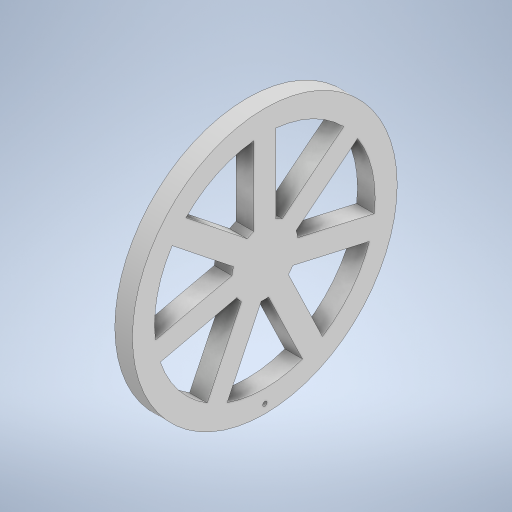
# Autodesk Inventor part: Langbektang houder
Saved by Autodesk Inventor 2023.2 (Build 272271000, 271)
## iProperties
Created: 2020-09-09
Part Number: Langbektang houder
Material: Generic
Document SubType Name: Modeling
Designer: nathan.bollaert
Density: 1 g/cm^3
Appearance: Default
Author: nathan.bollaert
Autodesk Inventor part; units mm, degrees
ref_plane "YZ Plane" through (0, 0, 0) normal (1, 0, 0) x (0, 1, 0)
ref_plane "XZ Plane" through (0, 0, 0) normal (0, 1, 0) x (-1, 0, 0)
ref_plane "XY Plane" through (0, 0, 0) normal (0, 0, 1) x (1, 0, 0)
sketch "Sketch1" plane through (0, 0, 0) normal (1, 0, 0) x (0, 1, 0)
  circle A0 centre (0, 0) radius 30
  dimension "d228" = 60
  constraints: 1 centre point, 1 coincident
  measures "d228" diameter of A0
extrude "Extrusion1" add sketch "Sketch1" along normal blind 4
sketch "Sketch2" plane through (4, 0, 0) normal (1, 0, 0) x (0, 0, -1)
  circle A0 centre (0, -28) radius 0.5
  point P0 (0, 0)
  dimension "d231" = 1
  dimension "d233" = 28
  constraints: 1 centre point, 1 vertical alignment
  measures "d231" diameter of A0
  measures "d233" distance of point (0, 0) A0.centre
hole "Hole1" at (4, -28, 0) direction (-1, 0, 0) diameter 1 end through all
sketch "Sketch3" plane through (4, 0, 0) normal (1, 0, 0) x (0, 0, -1)
  circle A0 centre (0, 0) radius 30 projected
  line L0 (-2.5, 25) -> (2.5, 25)
  line L1 (0, -42) -> (0, 42) projected
  circle A1 centre (0, 0) radius 7.5
  line L2 (2.5, 25) -> (2.5, 7.0711)
  line L3 (-2.5, 7.0711) -> (-2.5, 25)
  circle A2 centre (0, 0) radius 25
  line L4 (-17.9871, 17.5418) -> (-3.9697, 6.3633)
  line L5 (-21.1045, 13.6327) -> (-17.9871, 17.5418)
  line L6 (-7.0871, 2.4542) -> (-21.1045, 13.6327)
  line L7 (-24.9295, -3.1257) -> (-7.4501, 0.8639)
  line L8 (-23.8169, -8.0003) -> (-24.9295, -3.1257)
  line L9 (-6.3375, -4.0108) -> (-23.8169, -8.0003)
  line L10 (-13.0995, -21.4395) -> (-5.3204, -5.2861)
  line L11 (-8.5947, -23.6089) -> (-13.0995, -21.4395)
  line L12 (-0.8156, -7.4555) -> (-8.5947, -23.6089)
  line L13 (8.5947, -23.6089) -> (0.8156, -7.4555)
  line L14 (13.0995, -21.4395) -> (8.5947, -23.6089)
  line L15 (5.3204, -5.2861) -> (13.0995, -21.4395)
  line L16 (23.8169, -8.0003) -> (6.3375, -4.0108)
  line L17 (24.9295, -3.1257) -> (23.8169, -8.0003)
  line L18 (7.4501, 0.8639) -> (24.9295, -3.1257)
  line L19 (21.1045, 13.6327) -> (7.0871, 2.4542)
  line L20 (17.9871, 17.5418) -> (21.1045, 13.6327)
  line L21 (3.9697, 6.3633) -> (17.9871, 17.5418)
  point P0 (23.6947, -7.9725)
  point P1 (13.0451, -21.3266)
  point P2 (-8.5403, -23.496)
  point P3 (8.5403, -23.496)
  point P4 (0.8156, -7.4555)
  point P5 (-13.0451, -21.3266)
  point P6 (-23.6947, -7.9725)
  point P7 (-24.8073, -3.0978)
  point P8 (-7.4501, 0.8639)
  point P9 (-21.0065, 13.5545)
  point P10 (-17.8891, 17.4637)
  point P11 (-2.5, 24.8747)
  point P12 (17.8891, 17.4637)
  point P13 (2.5, 24.8747)
  point P14 (21.0065, 13.5545)
  point P15 (7.0871, 2.4542)
  point P16 (24.8073, -3.0978)
  dimension "d251" = 15
  dimension "d252" = 5
  dimension "d259" = 5
  dimension "d262" = 360
  constraints: 42 end point, 5 coincident, 2 centre point, 2 parallel, 2 point on circle, 1 tangent, 1 vertical, 51 other
  measures "d251" diameter of A1
  measures "d252" distance of L0.start L0.end
  measures "d259" radial gap between concentric circles of A0 A2
extrude "Extrusion2" cut sketch "Sketch3" against normal blind 4 contours A2 L12 A1 L1 | L1 A1 L13 A2 | A2 L21 A1 L2 | L3 A1 L4 A2 | L10 A2 L9 A1 | A1 L16 A2 L15 | L19 A2 L18 A1 | A1 L7 A2 L6
body "Solid5"
